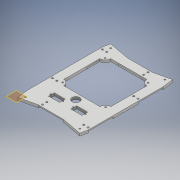
# Autodesk Inventor part: 3枚目
Saved by Autodesk Inventor 2018 (Build 220112000, 112)
## iProperties
Created: 2018-08-16
Part Number: 3枚目
Material: 一般
Document SubType Name: Modeling
Designer: shun2
Density: 1 g/cm^3
Appearance: 既定
Author: shun2
Autodesk Inventor part; units mm, degrees
ref_plane "YZ Plane" through (0, 0, 0) normal (1, 0, 0) x (0, 1, 0)
ref_plane "XZ Plane" through (0, 0, 0) normal (0, 1, 0) x (-1, 0, 0)
ref_plane "XY Plane" through (0, 0, 0) normal (0, 0, 1) x (1, 0, 0)
sketch "スケッチ1" plane through (0, 0, 0) normal (0, 0, 1) x (1, 0, 0)
  circle A0 centre (131.35, 19) radius 1.8
  circle A1 centre (122.35, 19) radius 1.8
  circle A2 centre (4.65, 71) radius 1.8
  circle A3 centre (13.65, 71) radius 1.8
  circle A4 centre (4.65, 175.7239) radius 1.8
  circle A5 centre (13.65, 175.7239) radius 1.8
  circle A6 centre (131.35, 123.7239) radius 1.8
  circle A7 centre (122.35, 123.7239) radius 1.8
  line L0 (0, 179.7239) -> (0, 23)
  line L1 (0, 23) -> (3, 0)
  line L2 (133, 0) -> (136, 15)
  line L3 (136, 15) -> (136, 171.7239)
  line L4 (136, 171.7239) -> (133, 194.7239)
  line L5 (0, 75) -> (18.3, 75)
  line L6 (18.3, 75) -> (18.3, 23)
  line L7 (18.3, 23) -> (0, 23)
  line L8 (0, 23) -> (0, 75)
  line L9 (0, 179.7239) -> (18.3, 179.7239)
  line L10 (18.3, 179.7239) -> (18.3, 127.7239)
  line L11 (18.3, 127.7239) -> (0, 127.7239)
  line L12 (0, 127.7239) -> (0, 179.7239)
  line L13 (46, 186.7239) -> (98, 186.7239)
  line L14 (98, 186.7239) -> (98, 168.4239)
  line L15 (98, 168.4239) -> (46, 168.4239)
  line L16 (46, 168.4239) -> (46, 186.7239)
  line L17 (117.7, 171.7239) -> (136, 171.7239)
  line L18 (136, 171.7239) -> (136, 119.7239)
  line L19 (136, 119.7239) -> (117.7, 119.7239)
  line L20 (117.7, 119.7239) -> (117.7, 171.7239)
  line L21 (117.7, 67) -> (136, 67)
  line L22 (136, 67) -> (136, 15)
  line L23 (136, 15) -> (117.7, 15)
  line L24 (117.7, 15) -> (117.7, 67)
  line L25 (38, 26.3) -> (90, 26.3)
  line L26 (90, 26.3) -> (90, 8)
  line L27 (90, 8.6122) -> (38, 8.6122)
  line L28 (38, 8) -> (38, 26.3)
  circle A8 centre (42, 12.65) radius 1.8
  circle A9 centre (42, 21.65) radius 1.8
  circle A10 centre (94, 182.0739) radius 1.8
  circle A11 centre (94, 173.0739) radius 1.8
  line L29 (3, 194.7239) -> (46, 186.7239)
  line L30 (98, 186.7239) -> (133, 194.7239)
  line L31 (3, 0) -> (38, 8)
  line L32 (38, 8) -> (90, 8)
  line L33 (90, 8) -> (133, 0)
  line L34 (46, 186.7239) -> (98, 186.7239)
  arc A12 (117.7, 160.734) -> (117.655, 160.7883) centre (112.29, 156.292) ccw
  arc A13 (117.655, 151.7957) -> (117.7, 151.8499) centre (112.29, 156.292) ccw
  line L35 (0, 179.7239) -> (3, 194.7239)
  circle A14 centre (11, 186.7239) radius 1.6
  circle A15 centre (125, 186.7239) radius 1.6
  circle A16 centre (11, 8) radius 1.6
  circle A17 centre (125, 8) radius 1.6
  line L36 (-39.2506, 184.5362) -> (-16.0026, 184.5362)
  line L37 (-16.0026, 184.5362) -> (-13.5186, 184.5362)
  line L38 (-13.5186, 184.5362) -> (-3.2973, 180.8977)
  line L39 (-3.1017, 181.4472) -> (-3.4929, 180.3481)
  line L40 (-3.4929, 180.3481) -> (0, 179.7239)
  line L41 (0, 179.7239) -> (-3.1017, 181.4472)
  line L42 (6.4, 186.7239) -> (15.6, 186.7239)
  line L43 (11, 182.1239) -> (11, 191.3239)
  line L44 (120.4, 186.7239) -> (129.6, 186.7239)
  line L45 (125, 182.1239) -> (125, 191.3239)
  line L46 (6.4, 8) -> (15.6, 8)
  line L47 (11, 3.4) -> (11, 12.6)
  line L48 (120.4, 8) -> (129.6, 8)
  line L49 (125, 3.4) -> (125, 12.6)
  line L50 (3, 194.7239) -> (0, 179.7239)
  line L51 (0, 23) -> (0, 179.7239)
  line L52 (3, 194.7239) -> (46, 186.7239)
  line L53 (46, 186.7239) -> (46, 168.4239)
  line L54 (46, 168.4239) -> (98, 168.4239)
  line L55 (98, 168.4239) -> (98, 186.7239)
  line L56 (133, 194.7239) -> (98, 186.7239)
  line L57 (133, 194.7239) -> (136, 171.7239)
  line L58 (136, 171.7239) -> (136, 15)
  line L59 (136, 15) -> (117.7, 15)
  line L60 (117.7, 15) -> (117.7, 67)
  line L61 (136, 67) -> (117.7, 67)
  line L62 (117.7, 119.7239) -> (136, 119.7239)
  line L63 (117.7, 119.7239) -> (117.7, 171.7239)
  line L64 (117.7, 171.7239) -> (136, 171.7239)
  line L65 (133, 0) -> (136, 15)
  line L66 (90, 8) -> (133, 0)
  line L67 (3, 0) -> (38, 8)
  line L68 (38, 26.3) -> (90, 26.3)
  line L69 (90, 26.3) -> (90, 8)
  line L70 (38, 8) -> (90, 8)
  line L71 (38, 26.3) -> (38, 8)
  line L72 (0, 23) -> (3, 0)
  line L73 (0, 179.7239) -> (18.3, 179.7239)
  line L74 (18.3, 179.7239) -> (18.3, 127.7239)
  line L75 (18.3, 127.7239) -> (0, 127.7239)
  line L76 (0, 127.7239) -> (0, 179.7239)
  line L77 (0, 75) -> (18.3, 75)
  line L78 (18.3, 75) -> (18.3, 23)
  line L79 (18.3, 23) -> (0, 23)
  line L80 (0, 23) -> (0, 75)
  line L81 (0, 127.7239) -> (0, 75)
  circle A18 centre (125, 186.7239) radius 1.6
  circle A19 centre (11, 186.7239) radius 1.6
  circle A20 centre (94, 182.0739) radius 1.8
  circle A21 centre (94, 182.0739) radius 1.8
  circle A22 centre (94, 173.0739) radius 1.8
  circle A23 centre (125, 186.7239) radius 1.6
  circle A24 centre (11, 186.7239) radius 1.6
  circle A25 centre (13.65, 175.7239) radius 1.8
  circle A26 centre (4.65, 175.7239) radius 1.8
  circle A27 centre (122.35, 123.7239) radius 1.8
  circle A28 centre (131.35, 123.7239) radius 1.8
  circle A29 centre (122.35, 19) radius 1.8
  circle A30 centre (131.35, 19) radius 1.8
  circle A31 centre (125, 8) radius 1.6
  circle A32 centre (42, 21.65) radius 1.8
  circle A33 centre (42, 12.65) radius 1.8
  circle A34 centre (4.65, 71) radius 1.8
  circle A35 centre (13.65, 71) radius 1.8
  circle A36 centre (11, 8) radius 1.6
  line L82 (117.7, 171.7239) -> (136, 171.7239)
  line L83 (136, 171.7239) -> (136, 119.7239)
  line L84 (136, 119.7239) -> (117.7, 119.7239)
  line L85 (117.7, 119.7239) -> (117.7, 171.7239)
  line L86 (117.7, 67) -> (136, 67)
  line L87 (136, 67) -> (136, 15)
  line L88 (136, 15) -> (117.7, 15)
  line L89 (117.7, 15) -> (117.7, 67)
  line L90 (33, 46.362) -> (56, 46.362)
  line L91 (56, 46.362) -> (56, 34.362)
  line L92 (56, 34.362) -> (33, 34.362)
  line L93 (33, 34.362) -> (33, 46.362)
  circle A37 centre (31.5, 40.362) radius 1.15
  circle A38 centre (57.5, 40.362) radius 1.15
  line L94 (80, 46.362) -> (103, 46.362)
  line L95 (103, 46.362) -> (103, 34.362)
  line L96 (103, 34.362) -> (80, 34.362)
  line L97 (80, 34.362) -> (80, 46.362)
  circle A39 centre (78.5, 40.362) radius 1.15
  circle A40 centre (104.5, 40.362) radius 1.15
  circle A41 centre (68, 56.6897) radius 8
  point P0 (0, 0)
  point P1 (-39.2506, 190.238)
  point P2 (-28.3321, 190.8402)
  dimension "d22" = 23
  dimension "d23" = 12
  dimension "d24" = 2.3
  dimension "d25" = 2.3
  dimension "d26" = 1.5
  dimension "d27" = 1.5
  dimension "d29" = 12
  dimension "d30" = 2.3
  dimension "d31" = 2.3
  dimension "d32" = 1.5
  dimension "d33" = 1.5
  dimension "d34" = 23
  dimension "d35" = 6
  dimension "d36" = 6
  dimension "d37" = 6
  dimension "d38" = 6
  dimension "d43" = 16
  dimension "d56" = 25.7498
  constraints: 196 end point, 42 centre point, 19 coincident, 14 concentric, 13 collinear, 13 perpendicular, 12 parallel, 6 horizontal, 4 point on circle, 1 vertical, 4 other
  measures "d22" distance of L91.end L92.end
  measures "d23" distance of L90.end L91.end
  measures "d24" diameter of A37
  measures "d25" diameter of A38
  measures "d26" distance from line of L93 A37.centre
  measures "d27" distance from line of L91 A38.centre
  measures "d29" distance of L95.start L95.end
  measures "d30" diameter of A39
  measures "d31" diameter of A40
  measures "d32" distance from line of L97 A39.centre
  measures "d33" distance from line of L95 A40.centre
  measures "d34" distance between parallel lines of L97 L95
  measures "d35" vertical distance of A39.centre L97.end
  measures "d36" vertical distance of A40.centre L95.start
  measures "d37" distance from line of A38.centre L90
  measures "d38" distance from line of A37.centre L90
  measures "d43" diameter of A41
  measures "d56" distance between parallel lines of L27 L92
ref_plane "作業平面1" through (0, 0, 5.5) normal (0, 0, 1) x (1, 0, 0)
sketch "スケッチ3" plane through (0, 0, 5.5) normal (0, 0, 1) x (1, 0, 0)
  circle A0 centre (131.35, 19) radius 1.8
  circle A1 centre (122.35, 19) radius 1.8
  circle A2 centre (4.65, 71) radius 1.8
  circle A3 centre (13.65, 71) radius 1.8
  circle A4 centre (4.65, 175.7239) radius 1.8
  circle A5 centre (13.65, 175.7239) radius 1.8
  circle A6 centre (131.35, 123.7239) radius 1.8
  circle A7 centre (122.35, 123.7239) radius 1.8
  line L0 (0, 179.7239) -> (0, 23)
  line L1 (0, 23) -> (3, 0)
  line L2 (133, 0) -> (136, 15)
  line L3 (136, 15) -> (136, 171.7239)
  line L4 (136, 171.7239) -> (133, 194.7239)
  line L5 (0, 75) -> (18.3, 75)
  line L6 (18.3, 75) -> (18.3, 23)
  line L7 (18.3, 23) -> (0, 23)
  line L8 (0, 23) -> (0, 75)
  line L9 (0, 179.7239) -> (18.3, 179.7239)
  line L10 (18.3, 179.7239) -> (18.3, 127.7239)
  line L11 (18.3, 127.7239) -> (0, 127.7239)
  line L12 (0, 127.7239) -> (0, 179.7239)
  line L13 (46, 186.7239) -> (98, 186.7239)
  line L14 (98, 186.7239) -> (98, 168.4239)
  line L15 (98, 168.4239) -> (46, 168.4239)
  line L16 (46, 168.4239) -> (46, 186.7239)
  line L17 (117.7, 171.7239) -> (136, 171.7239)
  line L18 (136, 171.7239) -> (136, 119.7239)
  line L19 (136, 119.7239) -> (117.7, 119.7239)
  line L20 (117.7, 119.7239) -> (117.7, 171.7239)
  line L21 (117.7, 67) -> (136, 67)
  line L22 (136, 67) -> (136, 15)
  line L23 (136, 15) -> (117.7, 15)
  line L24 (117.7, 15) -> (117.7, 67)
  line L25 (38, 26.3) -> (90, 26.3)
  line L26 (90, 26.3) -> (90, 8)
  line L27 (90, 8) -> (38, 8)
  line L28 (38, 8) -> (38, 26.3)
  circle A8 centre (42, 12.65) radius 1.8
  circle A9 centre (42, 21.65) radius 1.8
  circle A10 centre (94, 182.0739) radius 1.8
  circle A11 centre (94, 173.0739) radius 1.8
  line L29 (3, 194.7239) -> (46, 186.7239)
  line L30 (98, 186.7239) -> (133, 194.7239)
  line L31 (3, 0) -> (38, 8)
  line L32 (38, 8) -> (90, 8)
  line L33 (90, 8) -> (133, 0)
  line L34 (46, 186.7239) -> (98, 186.7239)
  circle A12 centre (23.71, 156.292) radius 1.59
  circle A13 centre (112.29, 156.292) radius 1.59
  circle A14 centre (112.29, 38.432) radius 1.59
  circle A15 centre (23.71, 38.432) radius 1.59
  arc A16 (105.29, 161.292) -> (112.29, 149.292) centre (112.8589, 157.6655) ccw
  arc A17 (23.71, 149.292) -> (30.71, 161.292) centre (23.1411, 157.6655) ccw
  arc A18 (117.7, 160.734) -> (117.655, 160.7883) centre (112.29, 156.292) ccw
  arc A19 (117.655, 151.7957) -> (117.7, 151.8499) centre (112.29, 156.292) ccw
  line L35 (30.71, 161.292) -> (105.29, 161.292)
  arc A20 (30.71, 33.432) -> (23.71, 45.432) centre (23.1411, 37.0584) ccw
  arc A21 (112.29, 45.432) -> (105.29, 33.432) centre (112.8589, 37.0584) ccw
  line L36 (23.71, 45.432) -> (23.71, 149.292)
  line L37 (112.29, 149.292) -> (112.29, 45.432)
  line L38 (16.4068, 85.862) -> (16.4068, 108.862)
  line L39 (16.4068, 108.862) -> (4.4068, 108.862)
  line L40 (4.4068, 108.862) -> (4.4068, 85.862)
  line L41 (4.4068, 85.862) -> (16.4068, 85.862)
  circle A22 centre (10.4068, 110.362) radius 1.15
  circle A23 centre (10.4068, 84.362) radius 1.15
  line L42 (0, 179.7239) -> (3, 194.7239)
  line L43 (30.71, 33.432) -> (105.29, 33.432)
  circle A24 centre (11, 186.7239) radius 1.6
  circle A25 centre (125, 186.7239) radius 1.6
  circle A26 centre (11, 8) radius 1.6
  circle A27 centre (125, 8) radius 1.6
  line L44 (-39.2506, 184.5362) -> (-16.0026, 184.5362)
  line L45 (-16.0026, 184.5362) -> (-13.5186, 184.5362)
  line L46 (-13.5186, 184.5362) -> (-3.2973, 180.8977)
  line L47 (-3.1017, 181.4472) -> (-3.4929, 180.3481)
  line L48 (-3.4929, 180.3481) -> (0, 179.7239)
  line L49 (0, 179.7239) -> (-3.1017, 181.4472)
  line L50 (6.4, 186.7239) -> (15.6, 186.7239)
  line L51 (11, 182.1239) -> (11, 191.3239)
  line L52 (120.4, 186.7239) -> (129.6, 186.7239)
  line L53 (125, 182.1239) -> (125, 191.3239)
  line L54 (6.4, 8) -> (15.6, 8)
  line L55 (11, 3.4) -> (11, 12.6)
  line L56 (120.4, 8) -> (129.6, 8)
  line L57 (125, 3.4) -> (125, 12.6)
  line L58 (0, 179.7239) -> (18.3, 179.7239) projected
  line L59 (18.3, 179.7239) -> (18.3, 127.7239) projected
  line L60 (0, 179.7239) -> (18.3, 179.7239)
  line L61 (18.3, 179.7239) -> (18.3, 127.7239)
  line L62 (18.3, 127.7239) -> (0, 127.7239)
  line L63 (0, 127.7239) -> (0, 179.7239)
  line L64 (46, 168.4239) -> (46, 186.7239) projected
  line L65 (98, 168.4239) -> (46, 168.4239) projected
  line L66 (46, 186.7239) -> (98, 186.7239)
  line L67 (98, 186.7239) -> (98, 168.4239)
  line L68 (98, 168.4239) -> (46, 168.4239)
  line L69 (46, 168.4239) -> (46, 186.7239)
  line L70 (136, 119.7239) -> (117.7, 119.7239)
  line L71 (117.7, 119.7239) -> (117.7, 171.7239)
  line L72 (117.7, 171.7239) -> (136, 171.7239)
  line L73 (136, 171.7239) -> (136, 119.7239)
  line L74 (117.7, 67) -> (136, 67)
  line L75 (136, 67) -> (136, 15)
  line L76 (136, 15) -> (117.7, 15)
  line L77 (117.7, 15) -> (117.7, 67)
  line L78 (38, 26.3) -> (90, 26.3) projected
  line L79 (90, 8) -> (38, 8)
  line L80 (38, 8) -> (38, 26.3)
  line L81 (38, 26.3) -> (90, 26.3)
  line L82 (90, 26.3) -> (90, 8)
  line L83 (18.3, 23) -> (0, 23)
  line L84 (0, 23) -> (0, 75)
  line L85 (0, 75) -> (18.3, 75)
  line L86 (18.3, 75) -> (18.3, 23)
  circle A28 centre (4.65, 175.7239) radius 1.8
  circle A29 centre (13.65, 175.7239) radius 1.8
  circle A30 centre (94, 182.0739) radius 1.8
  circle A31 centre (94, 173.0739) radius 1.8
  circle A32 centre (122.35, 123.7239) radius 1.8
  circle A33 centre (131.35, 123.7239) radius 1.8
  circle A34 centre (122.35, 19) radius 1.8
  circle A35 centre (131.35, 19) radius 1.8
  circle A36 centre (42, 21.65) radius 1.8
  circle A37 centre (42, 12.65) radius 1.8
  circle A38 centre (4.65, 71) radius 1.8
  circle A39 centre (13.65, 71) radius 1.8
  point P0 (0, 0)
  point P1 (-39.2506, 190.238)
  point P2 (-28.3321, 190.8402)
  constraints: 164 end point, 40 centre point, 12 coincident, 12 concentric, 12 parallel, 12 point on circle, 6 horizontal, 6 perpendicular
extrude "押し出し2" add sketch "スケッチ3" against normal blind 2.5 contours L9 L10 L11 L0 | L5 L6 L7 L0 | L13 L14 L15 L16 | L28 L25 L26 L27 | L3 L19 L20 L17 | L3 L23 L24 L21
ref_plane "作業平面2" through (0, 0, 5.5) normal (0, 0, 1) x (1, 0, 0)
sketch "スケッチ4" plane through (0, 0, 5.5) normal (0, 0, 1) x (1, 0, 0)
  line L0 (0, 179.7239) -> (0, 23) projected
  line L1 (0, 23) -> (18.3, 23) projected
  line L2 (136, 171.7239) -> (117.7, 171.7239) projected
  line L3 (29.8577, 168.0642) -> (105.8977, 168.0642)
  line L4 (117.3977, 156.5642) -> (117.3977, 80.8342)
  line L5 (105.8977, 69.3342) -> (29.8577, 69.3342)
  line L6 (18.3577, 80.8342) -> (18.3577, 156.5642)
  circle A0 centre (113.0141, 163.0973) radius 1.6
  circle A1 centre (113.0141, 74.1973) radius 1.6
  circle A2 centre (22.8441, 74.1973) radius 1.6
  circle A3 centre (22.8441, 163.0973) radius 1.6
  arc A4 (18.3577, 156.5642) -> (29.8577, 168.0642) centre (18.3577, 168.0642) ccw
  arc A5 (105.8977, 168.0642) -> (117.3977, 156.5642) centre (117.3977, 168.0642) ccw
  arc A6 (117.3977, 80.8342) -> (105.8977, 69.3342) centre (117.3977, 69.3342) ccw
  arc A7 (29.8577, 69.3342) -> (18.3577, 80.8342) centre (18.3577, 69.3342) ccw
  point P0 (0, 0)
  point P1 (18.0035, 68.7726)
  point P2 (67.8777, 118.6992)
  point P3 (68, 97.362)
  dimension "d14" = 3.2
  dimension "d15" = 3.2
  dimension "d16" = 3.2
  dimension "d17" = 3.2
  dimension "d44" = 23
  dimension "d45" = 23
  dimension "d46" = 23
  dimension "d47" = 23
  constraints: 8 centre point, 8 end point, 8 point on circle, 2 parallel, 1 horizontal, 1 perpendicular
  measures "d14" diameter of A0
  measures "d15" diameter of A1
  measures "d16" diameter of A2
  measures "d17" diameter of A3
  measures "d44" diameter of A4
  measures "d45" diameter of A5
  measures "d46" diameter of A6
  measures "d47" diameter of A7
extrude "押し出し3" add sketch "スケッチ1" along normal blind 5.5 contours L35 L29 L16 L15 L14 L30 L4 L17 L20 L19 L3 L21 L24 L23 L2 L33 L26 L25 L28 L31 L1 L7 L6 L5 L0 L11 L10 L9
extrude "押し出し4" cut sketch "スケッチ4" against normal blind 5.5
